Autodesk Fusion 360 part; units mm, degrees
(part 5 of 9)
  spline S19 degree 5 poles (-55.3327, -25.8588) (-55.3344, -25.8679) (-55.3377, -25.8861) (-55.3425, -25.9135) (-55.3488, -25.9499) (-55.3564, -25.9954) (-55.3637, -26.0408) (-55.3707, -26.0862) (-55.3774, -26.1315) (-55.3839, -26.1768) (-55.39, -26.222) (-55.3959, -26.2672) (-55.4014, -26.3123) (-55.4067, -26.3574) (-55.4116, -26.4024) (-55.4163, -26.4473) (-55.4207, -26.4922) (-55.4248, -26.537) (-55.4286, -26.5817) (-55.432, -26.6264) (-55.4352, -26.671) (-55.4381, -26.7155) (-55.4407, -26.7599) (-55.4429, -26.8043) (-55.4449, -26.8486) (-55.4466, -26.8928) (-55.4479, -26.9369) (-55.4489, -26.9809) (-55.4497, -27.0248) (-55.4501, -27.0687) (-55.4502, -27.1124) (-55.4499, -27.156) (-55.4494, -27.1996) (-55.4485, -27.243) (-55.4473, -27.2863) (-55.4458, -27.3296) (-55.444, -27.3727) (-55.4418, -27.4157) (-55.4393, -27.4585) (-55.4365, -27.5013) (-55.4333, -27.5439) (-55.4298, -27.5864) (-55.4259, -27.6288) (-55.4217, -27.671) (-55.4171, -27.7131) (-55.4122, -27.7551) (-55.4069, -27.7969) (-55.4013, -27.8386) (-55.3953, -27.8801) (-55.389, -27.9215) (-55.3822, -27.9627) (-55.3751, -28.0037) (-55.3676, -28.0445) (-55.3596, -28.0851) (-55.3512, -28.1256) (-55.3425, -28.1659) (-55.3333, -28.206) (-55.3238, -28.2459) (-55.3139, -28.2856) (-55.3036, -28.3251) (-55.2928, -28.3644) (-55.2814, -28.4033) (-55.2693, -28.442) (-55.2567, -28.4802) (-55.2434, -28.5182) (-55.2298, -28.556) (-55.2158, -28.5935) (-55.2015, -28.6309) (-55.1868, -28.668) (-55.1714, -28.7047) (-55.1546, -28.7406) (-55.1399, -28.7686) (-55.1278, -28.789) (-55.1193, -28.8024) (-55.115, -28.809) knots -1 -1 -1 -1 -1 -1 -0.98571429 -0.97142857 -0.95714286 -0.94285714 -0.92857143 -0.91428571 -0.9 -0.88571429 -0.87142857 -0.85714286 -0.84285714 -0.82857143 -0.81428571 -0.8 -0.78571429 -0.77142857 -0.75714286 -0.74285714 -0.72857143 -0.71428571 -0.7 -0.68571429 -0.67142857 -0.65714286 -0.64285714 -0.62857143 -0.61428571 -0.6 -0.58571429 -0.57142857 -0.55714286 -0.54285714 -0.52857143 -0.51428571 -0.5 -0.48571429 -0.47142857 -0.45714286 -0.44285714 -0.42857143 -0.41428571 -0.4 -0.38571429 -0.37142857 -0.35714286 -0.34285714 -0.32857143 -0.31428571 -0.3 -0.28571429 -0.27142857 -0.25714286 -0.24285714 -0.22857143 -0.21428571 -0.2 -0.18571429 -0.17142857 -0.15714286 -0.14285714 -0.12857143 -0.11428571 -0.1 -0.08571429 -0.07142857 -0.05714286 -0.04285714 -0.02857143 -0.01428571 0 0 0 0 0 0
  line L19 (-55.115, -28.809) -> (-54.3996, -29.8965)
  arc A39 (-54.5195, -30.5729) -> (-54.3996, -29.8965) centre (-54.8173, -30.1713) ccw
  arc A40 (-54.5195, -30.5729) -> (-55.4994, -31.422) centre (-49.427, -37.4399) ccw
  arc A41 (-56.1859, -31.4444) -> (-55.4994, -31.422) centre (-55.8545, -31.07) ccw
  line L20 (-56.1859, -31.4444) -> (-57.1606, -30.5815)
  spline S20 degree 5 poles (-57.1606, -30.5815) (-57.1665, -30.5763) (-57.1785, -30.566) (-57.197, -30.5511) (-57.2226, -30.5325) (-57.2558, -30.5109) (-57.2899, -30.4903) (-57.3245, -30.4705) (-57.3595, -30.4511) (-57.3947, -30.4319) (-57.4301, -30.413) (-57.4658, -30.3945) (-57.5019, -30.3765) (-57.5384, -30.3591) (-57.5754, -30.3422) (-57.6127, -30.3259) (-57.6503, -30.3101) (-57.6882, -30.2947) (-57.7264, -30.2796) (-57.7648, -30.2648) (-57.8034, -30.2504) (-57.8422, -30.2364) (-57.8813, -30.2227) (-57.9207, -30.2094) (-57.9603, -30.1965) (-58.0001, -30.184) (-58.0401, -30.1718) (-58.0804, -30.16) (-58.1208, -30.1485) (-58.1615, -30.1373) (-58.2023, -30.1265) (-58.2433, -30.116) (-58.2845, -30.1058) (-58.3259, -30.0959) (-58.3675, -30.0864) (-58.4092, -30.0772) (-58.4511, -30.0683) (-58.4932, -30.0597) (-58.5355, -30.0514) (-58.5779, -30.0435) (-58.6204, -30.0358) (-58.6632, -30.0285) (-58.706, -30.0215) (-58.749, -30.0147) (-58.7922, -30.0083) (-58.8355, -30.0022) (-58.879, -29.9963) (-58.9225, -29.9908) (-58.9663, -29.9855) (-59.0101, -29.9806) (-59.0541, -29.9759) (-59.0982, -29.9716) (-59.1424, -29.9675) (-59.1868, -29.9637) (-59.2312, -29.9603) (-59.2758, -29.9571) (-59.3205, -29.9542) (-59.3654, -29.9515) (-59.4103, -29.9492) (-59.4553, -29.9471) (-59.5005, -29.9454) (-59.5457, -29.9439) (-59.5911, -29.9427) (-59.6365, -29.9418) (-59.6821, -29.9411) (-59.7277, -29.9408) (-59.7734, -29.9407) (-59.8193, -29.9409) (-59.8652, -29.9414) (-59.9112, -29.9421) (-59.9573, -29.9431) (-59.9942, -29.9442) (-60.022, -29.9451) (-60.0405, -29.9458) (-60.0498, -29.9461) knots 0 0 0 0 0 0 0.01428571 0.02857143 0.04285714 0.05714286 0.07142857 0.08571429 0.1 0.11428571 0.12857143 0.14285714 0.15714286 0.17142857 0.18571429 0.2 0.21428571 0.22857143 0.24285714 0.25714286 0.27142857 0.28571429 0.3 0.31428571 0.32857143 0.34285714 0.35714286 0.37142857 0.38571429 0.4 0.41428571 0.42857143 0.44285714 0.45714286 0.47142857 0.48571429 0.5 0.51428571 0.52857143 0.54285714 0.55714286 0.57142857 0.58571429 0.6 0.61428571 0.62857143 0.64285714 0.65714286 0.67142857 0.68571429 0.7 0.71428571 0.72857143 0.74285714 0.75714286 0.77142857 0.78571429 0.8 0.81428571 0.82857143 0.84285714 0.85714286 0.87142857 0.88571429 0.9 0.91428571 0.92857143 0.94285714 0.95714286 0.97142857 0.98571429 1 1 1 1 1 1
  arc A42 (-60.0498, -29.9461) -> (-60.6564, -30.8901) centre (-49.427, -37.4399) ccw
  spline S21 degree 5 poles (-60.6564, -30.8901) (-60.6529, -30.8987) (-60.6458, -30.9158) (-60.6351, -30.9414) (-60.6207, -30.9755) (-60.6025, -31.0178) (-60.5841, -31.06) (-60.5655, -31.102) (-60.5466, -31.1437) (-60.5275, -31.1853) (-60.5082, -31.2267) (-60.4887, -31.2678) (-60.469, -31.3088) (-60.4491, -31.3496) (-60.4289, -31.3901) (-60.4086, -31.4304) (-60.388, -31.4705) (-60.3672, -31.5104) (-60.3462, -31.5501) (-60.325, -31.5896) (-60.3035, -31.6288) (-60.2819, -31.6678) (-60.26, -31.7066) (-60.238, -31.7451) (-60.2157, -31.7834) (-60.1932, -31.8215) (-60.1705, -31.8593) (-60.1475, -31.8969) (-60.1244, -31.9343) (-60.1011, -31.9714) (-60.0775, -32.0082) (-60.0537, -32.0448) (-60.0297, -32.0811) (-60.0055, -32.1172) (-59.9811, -32.153) (-59.9564, -32.1886) (-59.9316, -32.2238) (-59.9065, -32.2588) (-59.8812, -32.2935) (-59.8557, -32.328) (-59.83, -32.3621) (-59.804, -32.396) (-59.7779, -32.4295) (-59.7515, -32.4628) (-59.7249, -32.4957) (-59.6981, -32.5284) (-59.671, -32.5607) (-59.6438, -32.5927) (-59.6163, -32.6244) (-59.5886, -32.6558) (-59.5606, -32.6868) (-59.5325, -32.7174) (-59.504, -32.7477) (-59.4754, -32.7776) (-59.4465, -32.8071) (-59.4173, -32.8362) (-59.388, -32.865) (-59.3584, -32.8934) (-59.3286, -32.9215) (-59.2986, -32.9492) (-59.2682, -32.9764) (-59.2376, -33.003) (-59.2065, -33.0289) (-59.1752, -33.0543) (-59.1435, -33.0791) (-59.1116, -33.1035) (-59.0795, -33.1275) (-59.0473, -33.1512) (-59.0149, -33.1745) (-58.9821, -33.197) (-58.9486, -33.2182) (-58.921, -33.2337) (-58.8999, -33.2444) (-58.8855, -33.2511) (-58.8783, -33.2543) knots -1 -1 -1 -1 -1 -1 -0.98571429 -0.97142857 -0.95714286 -0.94285714 -0.92857143 -0.91428571 -0.9 -0.88571429 -0.87142857 -0.85714286 -0.84285714 -0.82857143 -0.81428571 -0.8 -0.78571429 -0.77142857 -0.75714286 -0.74285714 -0.72857143 -0.71428571 -0.7 -0.68571429 -0.67142857 -0.65714286 -0.64285714 -0.62857143 -0.61428571 -0.6 -0.58571429 -0.57142857 -0.55714286 -0.54285714 -0.52857143 -0.51428571 -0.5 -0.48571429 -0.47142857 -0.45714286 -0.44285714 -0.42857143 -0.41428571 -0.4 -0.38571429 -0.37142857 -0.35714286 -0.34285714 -0.32857143 -0.31428571 -0.3 -0.28571429 -0.27142857 -0.25714286 -0.24285714 -0.22857143 -0.21428571 -0.2 -0.18571429 -0.17142857 -0.15714286 -0.14285714 -0.12857143 -0.11428571 -0.1 -0.08571429 -0.07142857 -0.05714286 -0.04285714 -0.02857143 -0.01428571 0 0 0 0 0 0
  line L21 (-58.8783, -33.2543) -> (-57.6885, -33.7824)
  arc A43 (-57.4236, -34.4162) -> (-57.6885, -33.7824) centre (-57.8913, -34.2394) ccw
  circle A44 centre (-49.427, -37.4399) radius 2.5
  line L22 (-46.927, -37.4412) -> (-51.927, -37.4412)
  line L23 (-46.927, -37.4412) -> (-51.427, -37.4412)
  line L24 (-51.427, -37.4412) -> (-51.427, -38.9399)
  line L25 (-51.427, -37.4412) -> (-51.427, -35.9399)
  dimension "d69" = 4.5
  constraint coincident A44 L22.start
  constraint coincident A44 L22.end
  constraint horizontal L22
  constraint parallel L22 L23
  constraint coincident A44 L24.end
  constraint perpendicular L23 L24
  constraint coincident A44 L25.end
  constraint perpendicular L22 L25
  measures "d69" distance of L22.start L23.end
extrude "Extrude3'" add sketch "Sketch5" against normal blind 11.5 contours A44 L22 L25 | A44 L22 L24 sketch seen with x (1, 0, 0) y (0, 1, 0) z (0, 0, 1) at (-49.427, -37.4399, 0.3676) bodies 3 in component "Spur Gear (11 teeth)"
sketch "Sketch6" plane through (0, 0, -0.2907) normal (0, 0, -1) x (1, 0, 0)
  circle A0 centre (48.0648, 1.0985) radius 15
  arc A1 (66.2067, 10.6959) -> (65.7693, 9.3883) centre (66.6749, 9.8123) ccw
  line L0 (66.2067, 10.6959) -> (66.3384, 10.7657)
  spline S0 degree 5 poles (66.3384, 10.7657) (66.3471, 10.7703) (66.3642, 10.7797) (66.3895, 10.7944) (66.4225, 10.8151) (66.4628, 10.8428) (66.5024, 10.8717) (66.5415, 10.9013) (66.5803, 10.9314) (66.6191, 10.9618) (66.6576, 10.9924) (66.6959, 11.0234) (66.7339, 11.0549) (66.7716, 11.087) (66.8088, 11.1197) (66.8458, 11.1529) (66.8824, 11.1866) (66.9188, 11.2206) (66.955, 11.255) (66.9909, 11.2897) (67.0267, 11.3247) (67.0622, 11.36) (67.0975, 11.3957) (67.1325, 11.4317) (67.1673, 11.4681) (67.2019, 11.5048) (67.2362, 11.5418) (67.2704, 11.5792) (67.3043, 11.6168) (67.338, 11.6547) (67.3716, 11.6928) (67.4049, 11.7313) (67.438, 11.77) (67.4709, 11.809) (67.5036, 11.8483) (67.5361, 11.8879) (67.5684, 11.9277) (67.6005, 11.9677) (67.6324, 12.0081) (67.6641, 12.0486) (67.6956, 12.0894) (67.727, 12.1305) (67.7581, 12.1717) (67.7891, 12.2133) (67.8198, 12.255) (67.8504, 12.297) (67.8808, 12.3392) (67.911, 12.3817) (67.941, 12.4243) (67.9708, 12.4672) (68.0004, 12.5103) (68.0299, 12.5536) (68.0592, 12.5971) (68.0882, 12.6409) (68.1171, 12.6848) (68.1459, 12.729) (68.1744, 12.7733) (68.2028, 12.8179) (68.231, 12.8627) (68.259, 12.9076) (68.2868, 12.9528) (68.3144, 12.9981) (68.3419, 13.0437) (68.3692, 13.0894) (68.3963, 13.1353) (68.4232, 13.1814) (68.4499, 13.2277) (68.4765, 13.2742) (68.5029, 13.3209) (68.5291, 13.3677) (68.5551, 13.4148) (68.5758, 13.4525) (68.5913, 13.4809) (68.6015, 13.4999) (68.6067, 13.5094) knots 0 0 0 0 0 0 0.01428571 0.02857143 0.04285714 0.05714286 0.07142857 0.08571429 0.1 0.11428571 0.12857143 0.14285714 0.15714286 0.17142857 0.18571429 0.2 0.21428571 0.22857143 0.24285714 0.25714286 0.27142857 0.28571429 0.3 0.31428571 0.32857143 0.34285714 0.35714286 0.37142857 0.38571429 0.4 0.41428571 0.42857143 0.44285714 0.45714286 0.47142857 0.48571429 0.5 0.51428571 0.52857143 0.54285714 0.55714286 0.57142857 0.58571429 0.6 0.61428571 0.62857143 0.64285714 0.65714286 0.67142857 0.68571429 0.7 0.71428571 0.72857143 0.74285714 0.75714286 0.77142857 0.78571429 0.8 0.81428571 0.82857143 0.84285714 0.85714286 0.87142857 0.88571429 0.9 0.91428571 0.92857143 0.94285714 0.95714286 0.97142857 0.98571429 1 1 1 1 1 1
  arc A2 (68.6067, 13.5094) -> (67.8876, 14.6283) centre (48.0648, 1.0985) ccw
  spline S1 degree 5 poles (64.4496, 13.7048) (64.4573, 13.7108) (64.473, 13.7225) (64.4968, 13.7394) (64.5295, 13.7608) (64.5714, 13.786) (64.6141, 13.8099) (64.6573, 13.8332) (64.7008, 13.8561) (64.7445, 13.8787) (64.7884, 13.901) (64.8325, 13.923) (64.8769, 13.9445) (64.9218, 13.9654) (64.967, 13.9857) (65.0125, 14.0055) (65.0584, 14.0248) (65.1044, 14.0438) (65.1507, 14.0624) (65.1972, 14.0807) (65.2439, 14.0987) (65.2908, 14.1163) (65.3379, 14.1336) (65.3853, 14.1505) (65.4328, 14.1671) (65.4806, 14.1833) (65.5285, 14.1991) (65.5766, 14.2147) (65.625, 14.2299) (65.6734, 14.2448) (65.7221, 14.2595) (65.7709, 14.2738) (65.8199, 14.2878) (65.8691, 14.3015) (65.9184, 14.315) (65.9678, 14.3281) (66.0175, 14.341) (66.0672, 14.3535) (66.1172, 14.3658) (66.1672, 14.3778) (66.2175, 14.3895) (66.2678, 14.401) (66.3183, 14.4121) (66.3689, 14.423) (66.4197, 14.4337) (66.4706, 14.444) (66.5216, 14.4541) (66.5727, 14.464) (66.624, 14.4736) (66.6754, 14.4829) (66.7269, 14.4919) (66.7786, 14.5007) (66.8303, 14.5093) (66.8822, 14.5176) (66.9342, 14.5256) (66.9863, 14.5334) (67.0385, 14.5409) (67.0908, 14.5482) (67.1432, 14.5552) (67.1957, 14.562) (67.2484, 14.5686) (67.3011, 14.5749) (67.3539, 14.5809) (67.4069, 14.5868) (67.4599, 14.5923) (67.513, 14.5977) (67.5663, 14.6028) (67.6196, 14.6076) (67.673, 14.6123) (67.7265, 14.6166) (67.7801, 14.6208) (67.823, 14.6239) (67.8553, 14.6262) (67.8768, 14.6276) (67.8876, 14.6283) knots 0 0 0 0 0 0 0.01428571 0.02857143 0.04285714 0.05714286 0.07142857 0.08571429 0.1 0.11428571 0.12857143 0.14285714 0.15714286 0.17142857 0.18571429 0.2 0.21428571 0.22857143 0.24285714 0.25714286 0.27142857 0.28571429 0.3 0.31428571 0.32857143 0.34285714 0.35714286 0.37142857 0.38571429 0.4 0.41428571 0.42857143 0.44285714 0.45714286 0.47142857 0.48571429 0.5 0.51428571 0.52857143 0.54285714 0.55714286 0.57142857 0.58571429 0.6 0.61428571 0.62857143 0.64285714 0.65714286 0.67142857 0.68571429 0.7 0.71428571 0.72857143 0.74285714 0.75714286 0.77142857 0.78571429 0.8 0.81428571 0.82857143 0.84285714 0.85714286 0.87142857 0.88571429 0.9 0.91428571 0.92857143 0.94285714 0.95714286 0.97142857 0.98571429 1 1 1 1 1 1
  line L1 (64.4496, 13.7048) -> (64.3313, 13.614)
  arc A3 (62.9602, 13.7594) -> (64.3313, 13.614) centre (63.7221, 14.407) ccw
  arc A4 (62.9602, 13.7594) -> (62.7166, 14.0404) centre (48.0648, 1.0985) ccw
  arc A5 (62.7679, 15.4183) -> (62.7166, 14.0404) centre (63.4661, 14.7024) ccw
  line L2 (62.7679, 15.4183) -> (62.8746, 15.5224)
  spline S2 degree 5 poles (62.8746, 15.5224) (62.8816, 15.5292) (62.8954, 15.5431) (62.9156, 15.5643) (62.9414, 15.5935) (62.9723, 15.6314) (63.0021, 15.6703) (63.0312, 15.7097) (63.0601, 15.7495) (63.0887, 15.7896) (63.117, 15.8298) (63.145, 15.8704) (63.1726, 15.9113) (63.1997, 15.9527) (63.2263, 15.9946) (63.2524, 16.0368) (63.278, 16.0795) (63.3033, 16.1224) (63.3284, 16.1656) (63.3531, 16.209) (63.3775, 16.2526) (63.4016, 16.2965) (63.4255, 16.3407) (63.4489, 16.3851) (63.4721, 16.4299) (63.4949, 16.4748) (63.5174, 16.52) (63.5397, 16.5655) (63.5616, 16.6111) (63.5833, 16.657) (63.6047, 16.703) (63.6258, 16.7493) (63.6467, 16.7958) (63.6673, 16.8425) (63.6876, 16.8894) (63.7076, 16.9365) (63.7274, 16.9838) (63.7469, 17.0313) (63.7662, 17.079) (63.7852, 17.1268) (63.8039, 17.1749) (63.8224, 17.2231) (63.8407, 17.2715) (63.8587, 17.32) (63.8764, 17.3687) (63.8939, 17.4176) (63.9112, 17.4667) (63.9282, 17.5159) (63.945, 17.5653) (63.9615, 17.6149) (63.9778, 17.6646) (63.9939, 17.7144) (64.0097, 17.7644) (64.0253, 17.8146) (64.0406, 17.8649) (64.0558, 17.9154) (64.0706, 17.966) (64.0853, 18.0167) (64.0997, 18.0676) (64.1139, 18.1186) (64.1279, 18.1698) (64.1416, 18.2211) (64.1552, 18.2725) (64.1684, 18.3241) (64.1815, 18.3758) (64.1944, 18.4276) (64.207, 18.4796) (64.2194, 18.5317) (64.2316, 18.5839) (64.2435, 18.6362) (64.2552, 18.6887) (64.2645, 18.7307) (64.2713, 18.7623) (64.2758, 18.7834) (64.278, 18.794) knots 0 0 0 0 0 0 0.01428571 0.02857143 0.04285714 0.05714286 0.07142857 0.08571429 0.1 0.11428571 0.12857143 0.14285714 0.15714286 0.17142857 0.18571429 0.2 0.21428571 0.22857143 0.24285714 0.25714286 0.27142857 0.28571429 0.3 0.31428571 0.32857143 0.34285714 0.35714286 0.37142857 0.38571429 0.4 0.41428571 0.42857143 0.44285714 0.45714286 0.47142857 0.48571429 0.5 0.51428571 0.52857143 0.54285714 0.55714286 0.57142857 0.58571429 0.6 0.61428571 0.62857143 0.64285714 0.65714286 0.67142857 0.68571429 0.7 0.71428571 0.72857143 0.74285714 0.75714286 0.77142857 0.78571429 0.8 0.81428571 0.82857143 0.84285714 0.85714286 0.87142857 0.88571429 0.9 0.91428571 0.92857143 0.94285714 0.95714286 0.97142857 0.98571429 1 1 1 1 1 1
  arc A6 (64.278, 18.794) -> (63.2728, 19.665) centre (48.0648, 1.0985) ccw
  spline S3 degree 5 poles (60.2343, 17.8103) (60.24, 17.8182) (60.2517, 17.8338) (60.2699, 17.8568) (60.2951, 17.8865) (60.3283, 17.9225) (60.3625, 17.9575) (60.3974, 17.992) (60.4327, 18.0262) (60.4682, 18.0602) (60.504, 18.094) (60.5402, 18.1275) (60.5768, 18.1606) (60.6139, 18.1933) (60.6516, 18.2256) (60.6897, 18.2574) (60.7282, 18.2889) (60.7671, 18.32) (60.8063, 18.351) (60.8457, 18.3816) (60.8855, 18.412) (60.9255, 18.4421) (60.9658, 18.472) (61.0065, 18.5016) (61.0474, 18.5308) (61.0887, 18.5598) (61.1302, 18.5886) (61.172, 18.617) (61.2141, 18.6453) (61.2564, 18.6732) (61.299, 18.701) (61.3418, 18.7285) (61.3848, 18.7558) (61.4281, 18.7828) (61.4716, 18.8096) (61.5154, 18.8361) (61.5594, 18.8624) (61.6036, 18.8885) (61.6481, 18.9143) (61.6927, 18.9399) (61.7376, 18.9653) (61.7827, 18.9905) (61.828, 19.0154) (61.8735, 19.0402) (61.9192, 19.0647) (61.9651, 19.089) (62.0112, 19.113) (62.0575, 19.1369) (62.104, 19.1605) (62.1507, 19.1839) (62.1976, 19.2071) (62.2447, 19.2301) (62.2919, 19.2529) (62.3393, 19.2755) (62.387, 19.2978) (62.4347, 19.32) (62.4827, 19.3419) (62.5309, 19.3636) (62.5792, 19.3852) (62.6277, 19.4065) (62.6763, 19.4276) (62.7251, 19.4485) (62.7741, 19.4692) (62.8233, 19.4897) (62.8726, 19.51) (62.9221, 19.5301) (62.9717, 19.55) (63.0215, 19.5696) (63.0714, 19.5891) (63.1215, 19.6084) (63.1718, 19.6275) (63.2121, 19.6426) (63.2424, 19.6538) (63.2627, 19.6613) (63.2728, 19.665) knots 0 0 0 0 0 0 0.01428571 0.02857143 0.04285714 0.05714286 0.07142857 0.08571429 0.1 0.11428571 0.12857143 0.14285714 0.15714286 0.17142857 0.18571429 0.2 0.21428571 0.22857143 0.24285714 0.25714286 0.27142857 0.28571429 0.3 0.31428571 0.32857143 0.34285714 0.35714286 0.37142857 0.38571429 0.4 0.41428571 0.42857143 0.44285714 0.45714286 0.47142857 0.48571429 0.5 0.51428571 0.52857143 0.54285714 0.55714286 0.57142857 0.58571429 0.6 0.61428571 0.62857143 0.64285714 0.65714286 0.67142857 0.68571429 0.7 0.71428571 0.72857143 0.74285714 0.75714286 0.77142857 0.78571429 0.8 0.81428571 0.82857143 0.84285714 0.85714286 0.87142857 0.88571429 0.9 0.91428571 0.92857143 0.94285714 0.95714286 0.97142857 0.98571429 1 1 1 1 1 1
  line L3 (60.2343, 17.8103) -> (60.1464, 17.6898)
  arc A7 (58.7898, 17.443) -> (60.1464, 17.6898) centre (59.3384, 18.2791) ccw
  arc A8 (58.7898, 17.443) -> (58.477, 17.6441) centre (48.0648, 1.0985) ccw
  arc A9 (58.1379, 18.9806) -> (58.477, 17.6441) centre (59.0096, 18.4904) ccw
  line L4 (58.1379, 18.9806) -> (58.211, 19.1106)
  spline S4 degree 5 poles (58.211, 19.1106) (58.2158, 19.1191) (58.2252, 19.1362) (58.2385, 19.1623) (58.2551, 19.1976) (58.274, 19.2427) (58.2917, 19.2883) (58.3085, 19.3344) (58.325, 19.3807) (58.3411, 19.4272) (58.357, 19.4738) (58.3725, 19.5206) (58.3874, 19.5677) (58.4017, 19.615) (58.4154, 19.6627) (58.4285, 19.7106) (58.4412, 19.7587) (58.4533, 19.807) (58.4652, 19.8555) (58.4767, 19.9041) (58.4878, 19.9529) (58.4986, 20.0018) (58.509, 20.0509) (58.519, 20.1001) (58.5286, 20.1496) (58.5379, 20.1991) (58.5467, 20.2489) (58.5553, 20.2987) (58.5635, 20.3487) (58.5714, 20.3988) (58.5789, 20.4491) (58.5862, 20.4994) (58.5931, 20.5499) (58.5997, 20.6005) (58.6059, 20.6512) (58.6119, 20.7021) (58.6175, 20.753) (58.6229, 20.8041) (58.6279, 20.8552) (58.6327, 20.9065) (58.6371, 20.9579) (58.6413, 21.0094) (58.6452, 21.0609) (58.6488, 21.1126) (58.6521, 21.1643) (58.6551, 21.2162) (58.6578, 21.2681) (58.6603, 21.3201) (58.6625, 21.3723) (58.6644, 21.4245) (58.666, 21.4767) (58.6674, 21.5291) (58.6685, 21.5815) (58.6693, 21.6341) (58.6698, 21.6867) (58.6701, 21.7393) (58.6702, 21.7921) (58.6699, 21.8449) (58.6694, 21.8978) (58.6687, 21.9507) (58.6677, 22.0038) (58.6664, 22.0569) (58.6649, 22.11) (58.6631, 22.1633) (58.6611, 22.2165) (58.6588, 22.2699) (58.6563, 22.3233) (58.6535, 22.3768) (58.6505, 22.4303) (58.6472, 22.4839) (58.6437, 22.5375) (58.6407, 22.5805) (58.6383, 22.6127) (58.6367, 22.6342) (58.6358, 22.645) knots 0 0 0 0 0 0 0.01428571 0.02857143 0.04285714 0.05714286 0.07142857 0.08571429 0.1 0.11428571 0.12857143 0.14285714 0.15714286 0.17142857 0.18571429 0.2 0.21428571 0.22857143 0.24285714 0.25714286 0.27142857 0.28571429 0.3 0.31428571 0.32857143 0.34285714 0.35714286 0.37142857 0.38571429 0.4 0.41428571 0.42857143 0.44285714 0.45714286 0.47142857 0.48571429 0.5 0.51428571 0.52857143 0.54285714 0.55714286 0.57142857 0.58571429 0.6 0.61428571 0.62857143 0.64285714 0.65714286 0.67142857 0.68571429 0.7 0.71428571 0.72857143 0.74285714 0.75714286 0.77142857 0.78571429 0.8 0.81428571 0.82857143 0.84285714 0.85714286 0.87142857 0.88571429 0.9 0.91428571 0.92857143 0.94285714 0.95714286 0.97142857 0.98571429 1 1 1 1 1 1
  arc A10 (58.6358, 22.645) -> (57.426, 23.1975) centre (48.0648, 1.0985) ccw
  spline S5 degree 5 poles (55.033, 20.5619) (55.0363, 20.5711) (55.0432, 20.5894) (55.0541, 20.6166) (55.07, 20.6522) (55.0916, 20.696) (55.1146, 20.7393) (55.1384, 20.7822) (55.1626, 20.8249) (55.1871, 20.8676) (55.212, 20.9101) (55.2372, 20.9524) (55.263, 20.9945) (55.2894, 21.0364) (55.3164, 21.0779) (55.344, 21.1192) (55.3722, 21.1602) (55.4007, 21.2011) (55.4296, 21.2418) (55.4588, 21.2823) (55.4883, 21.3227) (55.5183, 21.3629) (55.5485, 21.4029) (55.5792, 21.4427) (55.6103, 21.4823) (55.6417, 21.5218) (55.6735, 21.561) (55.7055, 21.6001) (55.738, 21.6391) (55.7707, 21.6779) (55.8037, 21.7165) (55.837, 21.7549) (55.8706, 21.7932) (55.9046, 21.8313) (55.9388, 21.8693) (55.9733, 21.9071) (56.0081, 21.9447) (56.0432, 21.9822) (56.0786, 22.0195) (56.1142, 22.0567) (56.1501, 22.0937) (56.1863, 22.1305) (56.2227, 22.1672) (56.2594, 22.2038) (56.2963, 22.2402) (56.3336, 22.2764) (56.371, 22.3125) (56.4087, 22.3484) (56.4467, 22.3842) (56.4849, 22.4198) (56.5233, 22.4553) (56.562, 22.4906) (56.6009, 22.5258) (56.6401, 22.5608) (56.6795, 22.5956) (56.7191, 22.6304) (56.7589, 22.6649) (56.799, 22.6993) (56.8393, 22.7336) (56.8798, 22.7677) (56.9205, 22.8017) (56.9615, 22.8355) (57.0027, 22.8691) (57.044, 22.9027) (57.0856, 22.936) (57.1275, 22.9692) (57.1695, 23.0023) (57.2117, 23.0352) (57.2541, 23.068) (57.2968, 23.1006) (57.3396, 23.1331) (57.3741, 23.1589) (57.4, 23.1782) (57.4173, 23.1911) (57.426, 23.1975) knots 0 0 0 0 0 0 0.01428571 0.02857143 0.04285714 0.05714286 0.07142857 0.08571429 0.1 0.11428571 0.12857143 0.14285714 0.15714286 0.17142857 0.18571429 0.2 0.21428571 0.22857143 0.24285714 0.25714286 0.27142857 0.28571429 0.3 0.31428571 0.32857143 0.34285714 0.35714286 0.37142857 0.38571429 0.4 0.41428571 0.42857143 0.44285714 0.45714286 0.47142857 0.48571429 0.5 0.51428571 0.52857143 0.54285714 0.55714286 0.57142857 0.58571429 0.6 0.61428571 0.62857143 0.64285714 0.65714286 0.67142857 0.68571429 0.7 0.71428571 0.72857143 0.74285714 0.75714286 0.77142857 0.78571429 0.8 0.81428571 0.82857143 0.84285714 0.85714286 0.87142857 0.88571429 0.9 0.91428571 0.92857143 0.94285714 0.95714286 0.97142857 0.98571429 1 1 1 1 1 1
  line L5 (55.033, 20.5619) -> (54.9827, 20.4216)
  arc A11 (53.7506, 19.8026) -> (54.9827, 20.4216) centre (54.0414, 20.7593) ccw
  arc A12 (53.7506, 19.8026) -> (53.3938, 19.9073) centre (48.0648, 1.0985) ccw
  arc A13 (52.6919, 21.0942) -> (53.3938, 19.9073) centre (53.6664, 20.8695) ccw
  line L6 (52.6919, 21.0942) -> (52.7254, 21.2395)
  spline S6 degree 5 poles (52.7254, 21.2395) (52.7276, 21.249) (52.7318, 21.2681) (52.7373, 21.2968) (52.7432, 21.3354) (52.7486, 21.384) (52.7527, 21.4328) (52.7559, 21.4817) (52.7587, 21.5308) (52.7611, 21.5799) (52.7632, 21.6291) (52.7648, 21.6784) (52.7659, 21.7278) (52.7663, 21.7772) (52.766, 21.8268) (52.7651, 21.8764) (52.7636, 21.9262) (52.7617, 21.976) (52.7594, 22.0258) (52.7568, 22.0757) (52.7537, 22.1256) (52.7503, 22.1756) (52.7464, 22.2257) (52.7422, 22.2757) (52.7375, 22.3259) (52.7323, 22.376) (52.7269, 22.4262) (52.721, 22.4765) (52.7148, 22.5268) (52.7082, 22.5771) (52.7013, 22.6274) (52.6941, 22.6778) (52.6865, 22.7281) (52.6786, 22.7786) (52.6703, 22.829) (52.6617, 22.8795) (52.6528, 22.9299) (52.6435, 22.9804) (52.6339, 23.0309) (52.624, 23.0815) (52.6138, 23.132) (52.6033, 23.1826) (52.5925, 23.2331) (52.5814, 23.2837) (52.57, 23.3343) (52.5583, 23.3849) (52.5463, 23.4355) (52.534, 23.4861) (52.5214, 23.5367) (52.5085, 23.5874) (52.4954, 23.638) (52.4819, 23.6886) (52.4682, 23.7392) (52.4542, 23.7899) (52.4399, 23.8405) (52.4253, 23.8911) (52.4105, 23.9417) (52.3954, 23.9923) (52.38, 24.0429) (52.3644, 24.0935) (52.3485, 24.1441) (52.3323, 24.1947) (52.3159, 24.2453) (52.2992, 24.2959) (52.2822, 24.3464) (52.265, 24.397) (52.2475, 24.4475) (52.2298, 24.498) (52.2118, 24.5485) (52.1936, 24.599) (52.1751, 24.6495) (52.1601, 24.6899) (52.1487, 24.7202) (52.1411, 24.7403) (52.1373, 24.7504) knots 0 0 0 0 0 0 0.01428571 0.02857143 0.04285714 0.05714286 0.07142857 0.08571429 0.1 0.11428571 0.12857143 0.14285714 0.15714286 0.17142857 0.18571429 0.2 0.21428571 0.22857143 0.24285714 0.25714286 0.27142857 0.28571429 0.3 0.31428571 0.32857143 0.34285714 0.35714286 0.37142857 0.38571429 0.4 0.41428571 0.42857143 0.44285714 0.45714286 0.47142857 0.48571429 0.5 0.51428571 0.52857143 0.54285714 0.55714286 0.57142857 0.58571429 0.6 0.61428571 0.62857143 0.64285714 0.65714286 0.67142857 0.68571429 0.7 0.71428571 0.72857143 0.74285714 0.75714286 0.77142857 0.78571429 0.8 0.81428571 0.82857143 0.84285714 0.85714286 0.87142857 0.88571429 0.9 0.91428571 0.92857143 0.94285714 0.95714286 0.97142857 0.98571429 1 1 1 1 1 1
  arc A14 (52.1373, 24.7504) -> (50.8208, 24.9397) centre (48.0648, 1.0985) ccw
  spline S7 degree 5 poles (49.2673, 21.7367) (49.2679, 21.7465) (49.2693, 21.7659) (49.2721, 21.795) (49.2773, 21.8337) (49.2857, 21.8819) (49.2956, 21.9298) (49.3063, 21.9777) (49.3175, 22.0256) (49.329, 22.0734) (49.3409, 22.1212) (49.3532, 22.1689) (49.3661, 22.2166) (49.3796, 22.2642) (49.3938, 22.3116) (49.4087, 22.359) (49.4241, 22.4063) (49.44, 22.4536) (49.4562, 22.5007) (49.4728, 22.5479) (49.4898, 22.5949) (49.5072, 22.6419) (49.525, 22.6888) (49.5432, 22.7357) (49.5618, 22.7824) (49.5809, 22.8291) (49.6003, 22.8758) (49.6201, 22.9223) (49.6402, 22.9688) (49.6606, 23.0152) (49.6814, 23.0616) (49.7026, 23.1079) (49.7241, 23.1541) (49.7459, 23.2002) (49.768, 23.2463) (49.7905, 23.2923) (49.8133, 23.3382) (49.8364, 23.384) (49.8598, 23.4298) (49.8835, 23.4755) (49.9075, 23.5211) (49.9319, 23.5667) (49.9565, 23.6122) (49.9814, 23.6576) (50.0066, 23.7029) (50.0321, 23.7481) (50.0579, 23.7933) (50.0839, 23.8384) (50.1103, 23.8834) (50.1369, 23.9284) (50.1638, 23.9732) (50.1909, 24.018) (50.2184, 24.0627) (50.2461, 24.1073) (50.274, 24.1519) (50.3023, 24.1964) (50.3308, 24.2407) (50.3595, 24.2851) (50.3885, 24.3293) (50.4178, 24.3734) (50.4473, 24.4175) (50.4771, 24.4615) (50.5071, 24.5054) (50.5374, 24.5492) (50.5679, 24.5929) (50.5987, 24.6366) (50.6297, 24.6801) (50.6609, 24.7236) (50.6924, 24.767) (50.7241, 24.8103) (50.7561, 24.8535) (50.7818, 24.888) (50.8013, 24.9139) (50.8143, 24.9311) (50.8208, 24.9397) knots 0 0 0 0 0 0 0.01428571 0.02857143 0.04285714 0.05714286 0.07142857 0.08571429 0.1 0.11428571 0.12857143 0.14285714 0.15714286 0.17142857 0.18571429 0.2 0.21428571 0.22857143 0.24285714 0.25714286 0.27142857 0.28571429 0.3 0.31428571 0.32857143 0.34285714 0.35714286 0.37142857 0.38571429 0.4 0.41428571 0.42857143 0.44285714 0.45714286 0.47142857 0.48571429 0.5 0.51428571 0.52857143 0.54285714 0.55714286 0.57142857 0.58571429 0.6 0.61428571 0.62857143 0.64285714 0.65714286 0.67142857 0.68571429 0.7 0.71428571 0.72857143 0.74285714 0.75714286 0.77142857 0.78571429 0.8 0.81428571 0.82857143 0.84285714 0.85714286 0.87142857 0.88571429 0.9 0.91428571 0.92857143 0.94285714 0.95714286 0.97142857 0.98571429 1 1 1 1 1 1
  line L7 (49.2673, 21.7367) -> (49.2585, 21.5878)
  arc A15 (48.2507, 20.6468) -> (49.2585, 21.5878) centre (48.2602, 21.6467) ccw
  arc A16 (48.2507, 20.6468) -> (47.8788, 20.6468) centre (48.0648, 1.0985) ccw
  arc A17 (46.8711, 21.5878) -> (47.8788, 20.6468) centre (47.8693, 21.6467) ccw
  line L8 (46.8711, 21.5878) -> (46.8623, 21.7367)
  spline S8 degree 5 poles (46.8623, 21.7367) (46.8617, 21.7465) (46.8603, 21.7659) (46.8575, 21.795) (46.8523, 21.8337) (46.8438, 21.8819) (46.834, 21.9298) (46.8233, 21.9777) (46.8121, 22.0256) (46.8005, 22.0734) (46.7887, 22.1212) (46.7764, 22.1689) (46.7635, 22.2166) (46.75, 22.2642) (46.7357, 22.3116) (46.7209, 22.359) (46.7055, 22.4063) (46.6896, 22.4536) (46.6734, 22.5007) (46.6567, 22.5479) (46.6397, 22.5949) (46.6224, 22.6419) (46.6046, 22.6888) (46.5864, 22.7357) (46.5677, 22.7824) (46.5487, 22.8291) (46.5293, 22.8758) (46.5095, 22.9223) (46.4894, 22.9688) (46.4689, 23.0152) (46.4481, 23.0616) (46.427, 23.1079) (46.4055, 23.1541) (46.3837, 23.2002) (46.3615, 23.2463) (46.3391, 23.2923) (46.3163, 23.3382) (46.2932, 23.384) (46.2698, 23.4298) (46.246, 23.4755) (46.222, 23.5211) (46.1977, 23.5667) (46.1731, 23.6122) (46.1482, 23.6576) (46.123, 23.7029) (46.0975, 23.7481) (46.0717, 23.7933) (46.0456, 23.8384) (46.0193, 23.8834) (45.9927, 23.9284) (45.9658, 23.9732) (45.9386, 24.018) (45.9112, 24.0627) (45.8835, 24.1073) (45.8555, 24.1519) (45.8273, 24.1964) (45.7988, 24.2407) (45.77, 24.2851) (45.741, 24.3293) (45.7118, 24.3734) (45.6822, 24.4175) (45.6525, 24.4615) (45.6225, 24.5054) (45.5922, 24.5492) (45.5617, 24.5929) (45.5309, 24.6366) (45.4999, 24.6801) (45.4687, 24.7236) (45.4372, 24.767) (45.4054, 24.8103) (45.3735, 24.8535) (45.3477, 24.888) (45.3283, 24.9139) (45.3153, 24.9311) (45.3088, 24.9397) knots 0 0 0 0 0 0 0.01428571 0.02857143 0.04285714 0.05714286 0.07142857 0.08571429 0.1 0.11428571 0.12857143 0.14285714 0.15714286 0.17142857 0.18571429 0.2 0.21428571 0.22857143 0.24285714 0.25714286 0.27142857 0.28571429 0.3 0.31428571 0.32857143 0.34285714 0.35714286 0.37142857 0.38571429 0.4 0.41428571 0.42857143 0.44285714 0.45714286 0.47142857 0.48571429 0.5 0.51428571 0.52857143 0.54285714 0.55714286 0.57142857 0.58571429 0.6 0.61428571 0.62857143 0.64285714 0.65714286 0.67142857 0.68571429 0.7 0.71428571 0.72857143 0.74285714 0.75714286 0.77142857 0.78571429 0.8 0.81428571 0.82857143 0.84285714 0.85714286 0.87142857 0.88571429 0.9 0.91428571 0.92857143 0.94285714 0.95714286 0.97142857 0.98571429 1 1 1 1 1 1
  arc A18 (45.3088, 24.9397) -> (43.9923, 24.7504) centre (48.0648, 1.0985) ccw
  spline S9 degree 5 poles (43.4041, 21.2395) (43.4019, 21.249) (43.3978, 21.2681) (43.3923, 21.2968) (43.3864, 21.3354) (43.3809, 21.384) (43.3769, 21.4328) (43.3736, 21.4817) (43.3709, 21.5308) (43.3685, 21.5799) (43.3664, 21.6291) (43.3648, 21.6784) (43.3637, 21.7278) (43.3633, 21.7772) (43.3636, 21.8268) (43.3645, 21.8764) (43.3659, 21.9262) (43.3678, 21.976) (43.3701, 22.0258) (43.3728, 22.0757) (43.3758, 22.1256) (43.3793, 22.1756) (43.3831, 22.2257) (43.3874, 22.2757) (43.3921, 22.3259) (43.3972, 22.376) (43.4027, 22.4262) (43.4086, 22.4765) (43.4148, 22.5268) (43.4213, 22.5771) (43.4282, 22.6274) (43.4355, 22.6778) (43.4431, 22.7281) (43.451, 22.7786) (43.4593, 22.829) (43.4679, 22.8795) (43.4768, 22.9299) (43.4861, 22.9804) (43.4956, 23.0309) (43.5055, 23.0815) (43.5157, 23.132) (43.5262, 23.1826) (43.537, 23.2331) (43.5481, 23.2837) (43.5595, 23.3343) (43.5713, 23.3849) (43.5833, 23.4355) (43.5956, 23.4861) (43.6082, 23.5367) (43.621, 23.5874) (43.6342, 23.638) (43.6476, 23.6886) (43.6614, 23.7392) (43.6754, 23.7899) (43.6897, 23.8405) (43.7042, 23.8911) (43.719, 23.9417) (43.7342, 23.9923) (43.7495, 24.0429) (43.7652, 24.0935) (43.7811, 24.1441) (43.7972, 24.1947) (43.8137, 24.2453) (43.8304, 24.2959) (43.8473, 24.3464) (43.8646, 24.397) (43.882, 24.4475) (43.8998, 24.498) (43.9178, 24.5485) (43.936, 24.599) (43.9545, 24.6495) (43.9695, 24.6899) (43.9808, 24.7202) (43.9885, 24.7403) (43.9923, 24.7504) knots 0 0 0 0 0 0 0.01428571 0.02857143 0.04285714 0.05714286 0.07142857 0.08571429 0.1 0.11428571 0.12857143 0.14285714 0.15714286 0.17142857 0.18571429 0.2 0.21428571 0.22857143 0.24285714 0.25714286 0.27142857 0.28571429 0.3 0.31428571 0.32857143 0.34285714 0.35714286 0.37142857 0.38571429 0.4 0.41428571 0.42857143 0.44285714 0.45714286 0.47142857 0.48571429 0.5 0.51428571 0.52857143 0.54285714 0.55714286 0.57142857 0.58571429 0.6 0.61428571 0.62857143 0.64285714 0.65714286 0.67142857 0.68571429 0.7 0.71428571 0.72857143 0.74285714 0.75714286 0.77142857 0.78571429 0.8 0.81428571 0.82857143 0.84285714 0.85714286 0.87142857 0.88571429 0.9 0.91428571 0.92857143 0.94285714 0.95714286 0.97142857 0.98571429 1 1 1 1 1 1
  line L9 (43.4041, 21.2395) -> (43.4376, 21.0942)
  arc A19 (42.7358, 19.9073) -> (43.4376, 21.0942) centre (42.4632, 20.8695) ccw
  arc A20 (42.7358, 19.9073) -> (42.379, 19.8026) centre (48.0648, 1.0985) ccw
  arc A21 (41.1469, 20.4216) -> (42.379, 19.8026) centre (42.0881, 20.7593) ccw
  line L10 (41.1469, 20.4216) -> (41.0965, 20.5619)
  spline S10 degree 5 poles (41.0965, 20.5619) (41.0932, 20.5711) (41.0864, 20.5894) (41.0755, 20.6166) (41.0596, 20.6522) (41.0379, 20.696) (41.015, 20.7393) (40.9912, 20.7822) (40.967, 20.8249) (40.9424, 20.8676) (40.9176, 20.9101) (40.8923, 20.9524) (40.8666, 20.9945) (40.8401, 21.0364) (40.8131, 21.0779) (40.7855, 21.1192) (40.7574, 21.1602) (40.7289, 21.2011) (40.7, 21.2418) (40.6708, 21.2823) (40.6412, 21.3227) (40.6113, 21.3629) (40.581, 21.4029) (40.5503, 21.4427) (40.5193, 21.4823) (40.4879, 21.5218) (40.4561, 21.561) (40.424, 21.6001) (40.3916, 21.6391) (40.3589, 21.6779) (40.3259, 21.7165) (40.2926, 21.7549) (40.2589, 21.7932) (40.225, 21.8313) (40.1908, 21.8693) (40.1563, 21.9071) (40.1214, 21.9447) (40.0864, 21.9822) (40.051, 22.0195) (40.0154, 22.0567) (39.9795, 22.0937) (39.9433, 22.1305) (39.9069, 22.1672) (39.8702, 22.2038) (39.8332, 22.2402) (39.796, 22.2764) (39.7585, 22.3125) (39.7208, 22.3484) (39.6829, 22.3842) (39.6447, 22.4198) (39.6062, 22.4553) (39.5676, 22.4906) (39.5286, 22.5258) (39.4895, 22.5608) (39.4501, 22.5956) (39.4105, 22.6304) (39.3706, 22.6649) (39.3306, 22.6993) (39.2903, 22.7336) (39.2498, 22.7677) (39.209, 22.8017) (39.1681, 22.8355) (39.1269, 22.8691) (39.0855, 22.9027) (39.0439, 22.936) (39.0021, 22.9692) (38.9601, 23.0023) (38.9178, 23.0352) (38.8754, 23.068) (38.8328, 23.1006) (38.7899, 23.1331) (38.7555, 23.1589) (38.7296, 23.1782) (38.7122, 23.1911) (38.7036, 23.1975) knots 0 0 0 0 0 0 0.01428571 0.02857143 0.04285714 0.05714286 0.07142857 0.08571429 0.1 0.11428571 0.12857143 0.14285714 0.15714286 0.17142857 0.18571429 0.2 0.21428571 0.22857143 0.24285714 0.25714286 0.27142857 0.28571429 0.3 0.31428571 0.32857143 0.34285714 0.35714286 0.37142857 0.38571429 0.4 0.41428571 0.42857143 0.44285714 0.45714286 0.47142857 0.48571429 0.5 0.51428571 0.52857143 0.54285714 0.55714286 0.57142857 0.58571429 0.6 0.61428571 0.62857143 0.64285714 0.65714286 0.67142857 0.68571429 0.7 0.71428571 0.72857143 0.74285714 0.75714286 0.77142857 0.78571429 0.8 0.81428571 0.82857143 0.84285714 0.85714286 0.87142857 0.88571429 0.9 0.91428571 0.92857143 0.94285714 0.95714286 0.97142857 0.98571429 1 1 1 1 1 1
  arc A22 (38.7036, 23.1975) -> (37.4937, 22.645) centre (48.0648, 1.0985) ccw
  spline S11 degree 5 poles (37.9185, 19.1106) (37.9137, 19.1191) (37.9044, 19.1362) (37.891, 19.1623) (37.8745, 19.1976) (37.8556, 19.2427) (37.8379, 19.2883) (37.821, 19.3344) (37.8046, 19.3807) (37.7884, 19.4272) (37.7726, 19.4738) (37.7571, 19.5206) (37.7422, 19.5677) (37.7278, 19.615) (37.7142, 19.6627) (37.701, 19.7106) (37.6884, 19.7587) (37.6762, 19.807) (37.6644, 19.8555) (37.6529, 19.9041) (37.6417, 19.9529) (37.631, 20.0018) (37.6206, 20.0509) (37.6105, 20.1001) (37.6009, 20.1496) (37.5917, 20.1991) (37.5828, 20.2489) (37.5743, 20.2987) (37.5661, 20.3487) (37.5582, 20.3988) (37.5506, 20.4491) (37.5434, 20.4994) (37.5365, 20.5499) (37.5299, 20.6005) (37.5236, 20.6512) (37.5177, 20.7021) (37.512, 20.753) (37.5067, 20.8041) (37.5016, 20.8552) (37.4969, 20.9065) (37.4924, 20.9579) (37.4882, 21.0094) (37.4844, 21.0609) (37.4808, 21.1126) (37.4775, 21.1643) (37.4745, 21.2162) (37.4717, 21.2681) (37.4693, 21.3201) (37.4671, 21.3723) (37.4652, 21.4245) (37.4635, 21.4767) (37.4622, 21.5291) (37.4611, 21.5815) (37.4603, 21.6341) (37.4597, 21.6867) (37.4594, 21.7393) (37.4594, 21.7921) (37.4596, 21.8449) (37.4601, 21.8978) (37.4609, 21.9507) (37.4619, 22.0038) (37.4631, 22.0569) (37.4647, 22.11) (37.4664, 22.1633) (37.4685, 22.2165) (37.4707, 22.2699) (37.4733, 22.3233) (37.4761, 22.3768) (37.4791, 22.4303) (37.4824, 22.4839) (37.4859, 22.5375) (37.4889, 22.5805) (37.4913, 22.6127) (37.4929, 22.6342) (37.4937, 22.645) knots 0 0 0 0 0 0 0.01428571 0.02857143 0.04285714 0.05714286 0.07142857 0.08571429 0.1 0.11428571 0.12857143 0.14285714 0.15714286 0.17142857 0.18571429 0.2 0.21428571 0.22857143 0.24285714 0.25714286 0.27142857 0.28571429 0.3 0.31428571 0.32857143 0.34285714 0.35714286 0.37142857 0.38571429 0.4 0.41428571 0.42857143 0.44285714 0.45714286 0.47142857 0.48571429 0.5 0.51428571 0.52857143 0.54285714 0.55714286 0.57142857 0.58571429 0.6 0.61428571 0.62857143 0.64285714 0.65714286 0.67142857 0.68571429 0.7 0.71428571 0.72857143 0.74285714 0.75714286 0.77142857 0.78571429 0.8 0.81428571 0.82857143 0.84285714 0.85714286 0.87142857 0.88571429 0.9 0.91428571 0.92857143 0.94285714 0.95714286 0.97142857 0.98571429 1 1 1 1 1 1
  line L11 (37.9185, 19.1106) -> (37.9916, 18.9806)
  arc A23 (37.6526, 17.6441) -> (37.9916, 18.9806) centre (37.12, 18.4904) ccw
  arc A24 (37.6526, 17.6441) -> (37.3397, 17.443) centre (48.0648, 1.0985) ccw
  arc A25 (35.9832, 17.6898) -> (37.3397, 17.443) centre (36.7911, 18.2791) ccw
  line L12 (35.9832, 17.6898) -> (35.8953, 17.8103)
  spline S12 degree 5 poles (35.8953, 17.8103) (35.8895, 17.8182) (35.8778, 17.8338) (35.8597, 17.8568) (35.8344, 17.8865) (35.8013, 17.9225) (35.7671, 17.9575) (35.7322, 17.992) (35.6969, 18.0262) (35.6613, 18.0602) (35.6255, 18.094) (35.5894, 18.1275) (35.5528, 18.1606) (35.5156, 18.1933) (35.478, 18.2256) (35.4399, 18.2574) (35.4013, 18.2889) (35.3625, 18.32) (35.3233, 18.351) (35.2838, 18.3816) (35.2441, 18.412) (35.2041, 18.4421) (35.1637, 18.472) (35.1231, 18.5016) (35.0821, 18.5308) (35.0409, 18.5598) (34.9993, 18.5886) (34.9575, 18.617) (34.9155, 18.6453) (34.8732, 18.6732) (34.8306, 18.701) (34.7878, 18.7285) (34.7447, 18.7558) (34.7014, 18.7828) (34.6579, 18.8096) (34.6141, 18.8361) (34.5701, 18.8624) (34.5259, 18.8885) (34.4815, 18.9143) (34.4368, 18.9399) (34.3919, 18.9653) (34.3469, 18.9905) (34.3016, 19.0154) (34.2561, 19.0402) (34.2103, 19.0647) (34.1644, 19.089) (34.1183, 19.113) (34.072, 19.1369) (34.0255, 19.1605) (33.9788, 19.1839) (33.932, 19.2071) (33.8849, 19.2301) (33.8376, 19.2529) (33.7902, 19.2755) (33.7426, 19.2978) (33.6948, 19.32) (33.6468, 19.3419) (33.5987, 19.3636) (33.5504, 19.3852) (33.5019, 19.4065) (33.4532, 19.4276) (33.4044, 19.4485) (33.3554, 19.4692) (33.3063, 19.4897) (33.257, 19.51) (33.2075, 19.5301) (33.1579, 19.55) (33.1081, 19.5696) (33.0581, 19.5891) (33.008, 19.6084) (32.9578, 19.6275) (32.9174, 19.6426) (32.8871, 19.6538) (32.8669, 19.6613) (32.8568, 19.665) knots 0 0 0 0 0 0 0.01428571 0.02857143 0.04285714 0.05714286 0.07142857 0.08571429 0.1 0.11428571 0.12857143 0.14285714 0.15714286 0.17142857 0.18571429 0.2 0.21428571 0.22857143 0.24285714 0.25714286 0.27142857 0.28571429 0.3 0.31428571 0.32857143 0.34285714 0.35714286 0.37142857 0.38571429 0.4 0.41428571 0.42857143 0.44285714 0.45714286 0.47142857 0.48571429 0.5 0.51428571 0.52857143 0.54285714 0.55714286 0.57142857 0.58571429 0.6 0.61428571 0.62857143 0.64285714 0.65714286 0.67142857 0.68571429 0.7 0.71428571 0.72857143 0.74285714 0.75714286 0.77142857 0.78571429 0.8 0.81428571 0.82857143 0.84285714 0.85714286 0.87142857 0.88571429 0.9 0.91428571 0.92857143 0.94285714 0.95714286 0.97142857 0.98571429 1 1 1 1 1 1
  arc A26 (32.8568, 19.665) -> (31.8516, 18.794) centre (48.0648, 1.0985) ccw
  spline S13 degree 5 poles (33.2549, 15.5224) (33.2479, 15.5292) (33.2341, 15.5431) (33.214, 15.5643) (33.1881, 15.5935) (33.1573, 15.6314) (33.1275, 15.6703) (33.0983, 15.7097) (33.0695, 15.7495) (33.0409, 15.7896) (33.0125, 15.8298) (32.9845, 15.8704) (32.9569, 15.9113) (32.9298, 15.9527) (32.9033, 15.9946) (32.8772, 16.0368) (32.8515, 16.0795) (32.8262, 16.1224) (32.8012, 16.1656) (32.7765, 16.209) (32.752, 16.2526) (32.7279, 16.2965) (32.7041, 16.3407) (32.6806, 16.3851) (32.6575, 16.4299) (32.6346, 16.4748) (32.6121, 16.52) (32.5899, 16.5655) (32.5679, 16.6111) (32.5463, 16.657) (32.5248, 16.703) (32.5037, 16.7493) (32.4829, 16.7958) (32.4623, 16.8425) (32.442, 16.8894) (32.4219, 16.9365) (32.4021, 16.9838) (32.3826, 17.0313) (32.3634, 17.079) (32.3444, 17.1268) (32.3256, 17.1749) (32.3071, 17.2231) (32.2889, 17.2715) (32.2709, 17.32) (32.2531, 17.3687) (32.2356, 17.4176) (32.2184, 17.4667) (32.2014, 17.5159) (32.1846, 17.5653) (32.168, 17.6149) (32.1518, 17.6646) (32.1357, 17.7144) (32.1199, 17.7644) (32.1043, 17.8146) (32.0889, 17.8649) (32.0738, 17.9154) (32.0589, 17.966) (32.0443, 18.0167) (32.0298, 18.0676) (32.0156, 18.1186) (32.0017, 18.1698) (31.9879, 18.2211) (31.9744, 18.2725) (31.9611, 18.3241) (31.948, 18.3758) (31.9352, 18.4276) (31.9226, 18.4796) (31.9102, 18.5317) (31.898, 18.5839) (31.8861, 18.6362) (31.8743, 18.6887) (31.8651, 18.7307) (31.8583, 18.7623) (31.8538, 18.7834) (31.8516, 18.794) knots 0 0 0 0 0 0 0.01428571 0.02857143 0.04285714 0.05714286 0.07142857 0.08571429 0.1 0.11428571 0.12857143 0.14285714 0.15714286 0.17142857 0.18571429 0.2 0.21428571 0.22857143 0.24285714 0.25714286 0.27142857 0.28571429 0.3 0.31428571 0.32857143 0.34285714 0.35714286 0.37142857 0.38571429 0.4 0.41428571 0.42857143 0.44285714 0.45714286 0.47142857 0.48571429 0.5 0.51428571 0.52857143 0.54285714 0.55714286 0.57142857 0.58571429 0.6 0.61428571 0.62857143 0.64285714 0.65714286 0.67142857 0.68571429 0.7 0.71428571 0.72857143 0.74285714 0.75714286 0.77142857 0.78571429 0.8 0.81428571 0.82857143 0.84285714 0.85714286 0.87142857 0.88571429 0.9 0.91428571 0.92857143 0.94285714 0.95714286 0.97142857 0.98571429 1 1 1 1 1 1
  line L13 (33.2549, 15.5224) -> (33.3617, 15.4183)
  arc A27 (33.4129, 14.0404) -> (33.3617, 15.4183) centre (32.6634, 14.7024) ccw
  arc A28 (33.4129, 14.0404) -> (33.1694, 13.7594) centre (48.0648, 1.0985) ccw
  arc A29 (31.7982, 13.614) -> (33.1694, 13.7594) centre (32.4074, 14.407) ccw
  line L14 (31.7982, 13.614) -> (31.68, 13.7048)
  spline S14 degree 5 poles (31.68, 13.7048) (31.6722, 13.7108) (31.6566, 13.7225) (31.6327, 13.7394) (31.6001, 13.7608) (31.5582, 13.786) (31.5155, 13.8099) (31.4723, 13.8332) (31.4288, 13.8561) (31.3851, 13.8787) (31.3412, 13.901) (31.2971, 13.923) (31.2526, 13.9445) (31.2078, 13.9654) (31.1626, 13.9857) (31.117, 14.0055) (31.0712, 14.0248) (31.0251, 14.0438) (30.9788, 14.0624) (30.9323, 14.0807) (30.8856, 14.0987) (30.8387, 14.1163) (30.7916, 14.1336) (30.7443, 14.1505) (30.6968, 14.1671) (30.649, 14.1833) (30.601, 14.1991) (30.5529, 14.2147) (30.5046, 14.2299) (30.4561, 14.2448) (30.4075, 14.2595) (30.3586, 14.2738) (30.3097, 14.2878) (30.2605, 14.3015) (30.2112, 14.315) (30.1617, 14.3281) (30.1121, 14.341) (30.0623, 14.3535) (30.0124, 14.3658) (29.9623, 14.3778) (29.9121, 14.3895) (29.8618, 14.401) (29.8113, 14.4121) (29.7606, 14.423) (29.7099, 14.4337) (29.659, 14.444) (29.608, 14.4541) (29.5568, 14.464) (29.5056, 14.4736) (29.4542, 14.4829) (29.4026, 14.4919) (29.351, 14.5007) (29.2993, 14.5093) (29.2474, 14.5176) (29.1954, 14.5256) (29.1433, 14.5334) (29.0911, 14.5409) (29.0388, 14.5482) (28.9864, 14.5552) (28.9338, 14.562) (28.8812, 14.5686) (28.8285, 14.5749) (28.7756, 14.5809) (28.7227, 14.5868) (28.6697, 14.5923) (28.6165, 14.5977) (28.5633, 14.6028) (28.51, 14.6076) (28.4566, 14.6123) (28.4031, 14.6166) (28.3495, 14.6208) (28.3065, 14.6239) (28.2743, 14.6262) (28.2528, 14.6276) (28.242, 14.6283) knots 0 0 0 0 0 0 0.01428571 0.02857143 0.04285714 0.05714286 0.07142857 0.08571429 0.1 0.11428571 0.12857143 0.14285714 0.15714286 0.17142857 0.18571429 0.2 0.21428571 0.22857143 0.24285714 0.25714286 0.27142857 0.28571429 0.3 0.31428571 0.32857143 0.34285714 0.35714286 0.37142857 0.38571429 0.4 0.41428571 0.42857143 0.44285714 0.45714286 0.47142857 0.48571429 0.5 0.51428571 0.52857143 0.54285714 0.55714286 0.57142857 0.58571429 0.6 0.61428571 0.62857143 0.64285714 0.65714286 0.67142857 0.68571429 0.7 0.71428571 0.72857143 0.74285714 0.75714286 0.77142857 0.78571429 0.8 0.81428571 0.82857143 0.84285714 0.85714286 0.87142857 0.88571429 0.9 0.91428571 0.92857143 0.94285714 0.95714286 0.97142857 0.98571429 1 1 1 1 1 1
  arc A30 (28.242, 14.6283) -> (27.5229, 13.5094) centre (48.0648, 1.0985) ccw
  spline S15 degree 5 poles (29.7911, 10.7657) (29.7825, 10.7703) (29.7654, 10.7797) (29.74, 10.7944) (29.707, 10.8151) (29.6668, 10.8428) (29.6272, 10.8717) (29.5881, 10.9013) (29.5492, 10.9314) (29.5105, 10.9618) (29.472, 10.9924) (29.4336, 11.0234) (29.3956, 11.0549) (29.358, 11.087) (29.3207, 11.1197) (29.2838, 11.1529) (29.2471, 11.1866) (29.2108, 11.2206) (29.1746, 11.255) (29.1386, 11.2897) (29.1029, 11.3247) (29.0674, 11.36) (29.0321, 11.3957) (28.997, 11.4317) (28.9622, 11.4681) (28.9277, 11.5048) (28.8933, 11.5418) (28.8592, 11.5792) (28.8252, 11.6168) (28.7915, 11.6547) (28.758, 11.6928) (28.7247, 11.7313) (28.6916, 11.77) (28.6587, 11.809) (28.626, 11.8483) (28.5935, 11.8879) (28.5612, 11.9277) (28.5291, 11.9677) (28.4972, 12.0081) (28.4654, 12.0486) (28.4339, 12.0894) (28.4026, 12.1305) (28.3715, 12.1717) (28.3405, 12.2133) (28.3097, 12.255) (28.2792, 12.297) (28.2488, 12.3392) (28.2186, 12.3817) (28.1886, 12.4243) (28.1588, 12.4672) (28.1291, 12.5103) (28.0997, 12.5536) (28.0704, 12.5971) (28.0413, 12.6409) (28.0124, 12.6848) (27.9837, 12.729) (27.9551, 12.7733) (27.9268, 12.8179) (27.8986, 12.8627) (27.8706, 12.9076) (27.8428, 12.9528) (27.8151, 12.9981) (27.7877, 13.0437) (27.7604, 13.0894) (27.7333, 13.1353) (27.7064, 13.1814) (27.6796, 13.2277) (27.6531, 13.2742) (27.6267, 13.3209) (27.6004, 13.3677) (27.5744, 13.4148) (27.5537, 13.4525) (27.5383, 13.4809) (27.528, 13.4999) (27.5229, 13.5094) knots 0 0 0 0 0 0 0.01428571 0.02857143 0.04285714 0.05714286 0.07142857 0.08571429 0.1 0.11428571 0.12857143 0.14285714 0.15714286 0.17142857 0.18571429 0.2 0.21428571 0.22857143 0.24285714 0.25714286 0.27142857 0.28571429 0.3 0.31428571 0.32857143 0.34285714 0.35714286 0.37142857 0.38571429 0.4 0.41428571 0.42857143 0.44285714 0.45714286 0.47142857 0.48571429 0.5 0.51428571 0.52857143 0.54285714 0.55714286 0.57142857 0.58571429 0.6 0.61428571 0.62857143 0.64285714 0.65714286 0.67142857 0.68571429 0.7 0.71428571 0.72857143 0.74285714 0.75714286 0.77142857 0.78571429 0.8 0.81428571 0.82857143 0.84285714 0.85714286 0.87142857 0.88571429 0.9 0.91428571 0.92857143 0.94285714 0.95714286 0.97142857 0.98571429 1 1 1 1 1 1
  line L15 (29.7911, 10.7657) -> (29.9229, 10.6959)
  arc A31 (30.3603, 9.3883) -> (29.9229, 10.6959) centre (29.4546, 9.8123) ccw
  arc A32 (30.3603, 9.3883) -> (30.2058, 9.05) centre (48.0648, 1.0985) ccw
  arc A33 (28.9311, 8.5242) -> (30.2058, 9.05) centre (29.2922, 9.4567) ccw
  line L16 (28.9311, 8.5242) -> (28.792, 8.5781)
  spline S16 degree 5 poles (28.792, 8.5781) (28.7829, 8.5816) (28.7646, 8.5884) (28.737, 8.5979) (28.6996, 8.6093) (28.6523, 8.6216) (28.6046, 8.6326) (28.5566, 8.6427) (28.5084, 8.6524) (28.4601, 8.6618) (28.4117, 8.6708) (28.3632, 8.6795) (28.3145, 8.6876) (28.2656, 8.695) (28.2165, 8.7018) (28.1672, 8.708) (28.1178, 8.7136) (28.0682, 8.7188) (28.0186, 8.7236) (27.9688, 8.7281) (27.9189, 8.7322) (27.869, 8.7359) (27.8189, 8.7392) (27.7687, 8.7421) (27.7184, 8.7446) (27.6681, 8.7466) (27.6176, 8.7483) (27.567, 8.7497) (27.5164, 8.7507) (27.4656, 8.7514) (27.4148, 8.7517) (27.364, 8.7517) (27.313, 8.7514) (27.262, 8.7507) (27.2109, 8.7497) (27.1597, 8.7483) (27.1085, 8.7467) (27.0572, 8.7447) (27.0058, 8.7424) (26.9544, 8.7398) (26.9029, 8.7369) (26.8514, 8.7337) (26.7998, 8.7302) (26.7481, 8.7264) (26.6964, 8.7223) (26.6447, 8.7179) (26.5929, 8.7133) (26.541, 8.7083) (26.4891, 8.703) (26.4372, 8.6975) (26.3852, 8.6917) (26.3332, 8.6856) (26.2811, 8.6792) (26.229, 8.6725) (26.1769, 8.6656) (26.1247, 8.6584) (26.0725, 8.6509) (26.0202, 8.6432) (25.968, 8.6351) (25.9157, 8.6269) (25.8633, 8.6183) (25.8109, 8.6095) (25.7585, 8.6004) (25.7061, 8.5911) (25.6536, 8.5815) (25.6012, 8.5717) (25.5487, 8.5616) (25.4961, 8.5512) (25.4436, 8.5406) (25.391, 8.5297) (25.3384, 8.5186) (25.2963, 8.5095) (25.2647, 8.5026) (25.2437, 8.4979) (25.2332, 8.4955) knots 0 0 0 0 0 0 0.01428571 0.02857143 0.04285714 0.05714286 0.07142857 0.08571429 0.1 0.11428571 0.12857143 0.14285714 0.15714286 0.17142857 0.18571429 0.2 0.21428571 0.22857143 0.24285714 0.25714286 0.27142857 0.28571429 0.3 0.31428571 0.32857143 0.34285714 0.35714286 0.37142857 0.38571429 0.4 0.41428571 0.42857143 0.44285714 0.45714286 0.47142857 0.48571429 0.5 0.51428571 0.52857143 0.54285714 0.55714286 0.57142857 0.58571429 0.6 0.61428571 0.62857143 0.64285714 0.65714286 0.67142857 0.68571429 0.7 0.71428571 0.72857143 0.74285714 0.75714286 0.77142857 0.78571429 0.8 0.81428571 0.82857143 0.84285714 0.85714286 0.87142857 0.88571429 0.9 0.91428571 0.92857143 0.94285714 0.95714286 0.97142857 0.98571429 1 1 1 1 1 1
  arc A34 (25.2332, 8.4955) -> (24.8584, 7.2194) centre (48.0648, 1.0985) ccw